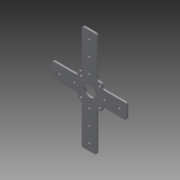
# Autodesk Inventor part: Plate 2
Saved by Autodesk Inventor 2014 (Build 180170000, 170)
## iProperties
Created: 2014-01-07
Part Number: Plate 2
Material: Generic
Document SubType Name: Modeling
Designer: Andrew Toennies
Density: 1 g/cm^3
Appearance: Default
Author: Andrew Toennies
Autodesk Inventor part; units mm, degrees
ref_plane "YZ Plane" through (0, 0, 0) normal (1, 0, 0) x (0, 1, 0)
ref_plane "XZ Plane" through (0, 0, 0) normal (0, 1, 0) x (-1, 0, 0)
ref_plane "XY Plane" through (0, 0, 0) normal (0, 0, 1) x (1, 0, 0)
sketch "Sketch1" plane through (0, 0, 0) normal (0, 0, 1) x (1, 0, 0)
  line L0 (127, 0) -> (127, -25.4)
  line L1 (0, -25.4) -> (0, 0)
  line L2 (127, -25.4) -> (85.6615, -25.4)
  line L3 (44.3865, 7.9375) -> (44.3865, 0)
  line L4 (44.3865, -25.4) -> (44.3865, -33.3375)
  line L5 (85.6615, 0) -> (127, 0)
  line L6 (85.6615, -33.3375) -> (85.6615, -25.4)
  line L7 (85.6615, 0) -> (85.6615, 7.9375)
  circle A0 centre (114.3, -12.7) radius 2.0828
  circle A1 centre (12.7, -12.7) radius 2.0828
  line L8 (80.899, 3.175) -> (49.149, 3.175) construction
  line L9 (49.149, 3.175) -> (49.149, -28.575) construction
  line L10 (49.149, -28.575) -> (80.899, -28.575) construction
  line L11 (80.899, -28.575) -> (80.899, 3.175) construction
  circle A2 centre (80.899, 3.175) radius 2.3876
  circle A3 centre (80.899, -28.575) radius 2.3876
  circle A4 centre (49.149, 3.175) radius 2.3876
  circle A5 centre (49.149, -28.575) radius 2.3876
  circle A6 centre (65.024, -12.7) radius 9.525
  line L12 (44.3865, 0) -> (0, 0)
  line L13 (0, -25.4) -> (44.3865, -25.4)
  line L14 (76.2, 7.9375) -> (76.2, 76.2)
  line L15 (76.2, 76.2) -> (50.8, 76.2)
  line L16 (50.8, 76.2) -> (50.8, 7.9375)
  line L17 (50.8, -33.3375) -> (50.8, -101.6)
  line L18 (50.8, -101.6) -> (76.2, -101.6)
  line L19 (76.2, -101.6) -> (76.2, -33.3375)
  line L20 (85.6615, 7.9375) -> (76.2, 7.9375)
  line L21 (50.8, 7.9375) -> (44.3865, 7.9375)
  line L22 (44.3865, -33.3375) -> (50.8, -33.3375)
  line L23 (76.2, -33.3375) -> (85.6615, -33.3375)
  circle A7 centre (63.5, 12.7) radius 2.0828
  circle A8 centre (63.5, -38.1) radius 2.0828
  circle A9 centre (63.5, 38.1) radius 2.0828
  circle A10 centre (63.5, 63.5) radius 2.0828
  circle A11 centre (63.5, -63.5) radius 2.0828
  circle A12 centre (63.5, -88.9) radius 2.0828
  circle A13 centre (88.9, -12.7) radius 2.0828
  circle A14 centre (38.1, -12.7) radius 2.0828
  dimension "d12" = 25.4
  dimension "d13" = 127
  dimension "d14" = 41.275
  dimension "d15" = 4.1656
  dimension "d16" = 4.1656
  dimension "d17" = 31.75
  dimension "d18" = 31.75
  dimension "d19" = 4.7625
  dimension "d20" = 12.7
  dimension "d21" = 12.7
  dimension "d22" = 12.7
  dimension "d23" = 4.7752
  dimension "d24" = 31.75
  dimension "d25" = 31.75
  dimension "d26" = 19.05
  dimension "d27" = 20.6375
  dimension "d28" = 61.976
  dimension "d29" = 12.7
  dimension "d30" = 25.4
  dimension "d31" = 50.8
  dimension "d32" = 76.2
  dimension "d33" = 25.4
  dimension "d34" = 76.2
  dimension "d35" = 41.275
  dimension "d36" = 4.7625
  dimension "d37" = 20.6375
  dimension "d38" = 4.1656
  dimension "d39" = 4.1656
  dimension "d40" = 12.7
  dimension "d41" = 12.7
  dimension "d42" = 25.4
  dimension "d43" = 12.7
  dimension "d44" = 12.7
  dimension "d45" = 25.4
  dimension "d53" = 25.4
  dimension "d60" = 25.4
  constraints: 48 end point, 16 parallel, 15 centre point, 12 perpendicular, 9 collinear, 7 horizontal, 3 vertical, 2 coincident, 18 other
  measures "d12" distance of L0.start L0.end
  measures "d13" distance of L0.end L1.start
  measures "d14" distance of L22.start L6.start
  measures "d15" diameter of A0
  measures "d16" diameter of A1
  measures "d17" distance of L10.end L8.start
  measures "d18" distance of L10.start L10.end
  measures "d19" distance between parallel lines of L7 L11
  measures "d20" distance from line of L0 A0.centre
  measures "d21" distance from line of L2 A0.centre
  measures "d22" distance from line of A1.centre L1
  measures "d23" diameter of A2
  measures "d24" distance of A2.centre A3.centre
  measures "d25" distance of A2.centre A4.centre
  measures "d26" diameter of A6
  measures "d27" distance from line of L7 A6.centre
  measures "d28" distance from line of L0 A6.centre
  measures "d29" distance from line of L12 A1.centre
  measures "d30" distance of L14.end L15.end
  measures "d31" distance between parallel lines of L16 L1
  measures "d32" distance between parallel lines of L12 L15
  measures "d33" distance of L17.end L19.start
  measures "d34" distance between parallel lines of L18 L13
  measures "d35" distance between parallel lines of L21 L22
  measures "d36" distance between parallel lines of L23 L10
  measures "d37" distance from line of L23 A6.centre
  measures "d38" diameter of A7
  measures "d39" diameter of A8
  measures "d40" distance from line of L14 A7.centre
  measures "d41" distance from line of L12 A7.centre
  measures "d42" distance of A7.centre A9.centre
  measures "d43" distance from line of L19 A8.centre
  measures "d44" distance from line of A8.centre L2
  measures "d45" distance of A8.centre A11.centre
  measures "d53" distance of A0.centre A13.centre
  measures "d60" distance of A1.centre A14.centre
extrude "Extrusion1" add sketch "Sketch1" along normal blind 3.175
fillet "Fillet1" radius 3.175 20 edges at (76.2, 7.9375, 1.5875) (85.6615, 7.9375, 1.5875) (85.6615, 0, 1.5875) (127, 0, 1.5875) (127, -25.4, 1.5875) (85.6615, -33.3375, 1.5875) (85.6615, -25.4, 1.5875) (76.2, -33.3375, 1.5875) (76.2, -101.6, 1.5875) (50.8, -101.6, 1.5875) (50.8, -33.3375, 1.5875) (44.3865, -33.3375, 1.5875) (44.3865, -25.4, 1.5875) (0, -25.4, 1.5875) (0, 0, 1.5875) (44.3865, 0, 1.5875) (50.8, 7.9375, 1.5875) (44.3865, 7.9375, 1.5875) (76.2, 76.2, 1.5875) (50.8, 76.2, 1.5875)
body "Solid1"
